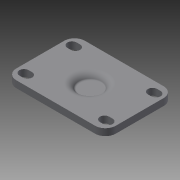
# Autodesk Inventor part: 2SS-TP
Saved by Autodesk Inventor 2014 SP2 (Build 180246200, 246)
## iProperties
Created: 2018-12-09
Part Number: 2SS-TP
Material: Generic
Catalog Web Link: www.cadenas.de
Description: 2 Series Stainless_Steel Top Plate-Capacitiy up to 325 lbs Each
Vendor: COLSONGROUP
Document SubType Name: Modeling
Designer: psadmin
Manufacturer: COLSONGROUP
Mass: 34.703 g
Surface Area: 138.104 cm^2
Volume: 34.703 cm^3
Density: 1 g/cm^3
Appearance: PSOLRGB-175-175-175
Category: PARTsolutions
Company: COLSONGROUP
Title: 2SS-TP
Author: Cadenas PARTsolutions
Comments: Capacitiy up to 325 lbs Each
PSOL_IDENT_0: {$CADENAS_DATA\23d-libs\colsongroup\colson\casters\2_series_stainless_steel\2_series_stainless_steel
PSOL_IDENT_1: _top_plate.prj},180 {VTYP=3D},{NB=2SS-TP},{LINA=2SS-TP},{NN=2 Series Stainless_Steel Top Plate},{DAT
PSOL_IDENT_2: E=13.07.2017 07:15:59},{GEOMDATE=03.02.2017 08:04:00},{VERSION=},{LINEID=40},{WBVAR=},{WBNUMERIC=}
PSOL_IDENT_3: {NB=2SS-TP},{LINA=2SS-TP},{KT=DUMMY},{PN=2SS-TP},{MO=TPS},{HEIGHT=2.50000000},{WIDTH=3.62500000},{HD
PSOL_IDENT_4: Y1=2.81250000},{HDY2=3.06250000},{HDX1=1.75000000},{THK=0.250},{HR=0.170}
NN: 2 Series Stainless_Steel Top Plate
NT: Capacitiy up to 325 lbs Each
NB: 2SS-TP
NBSYN: $PN.
LINA: 2SS-TP
PN: 2SS-TP
MO: TPS
HEIGHT: 2.5
WIDTH: 3.625
HDY1: 2.8125
HDY2: 3.0625
HDX1: 1.75
THK: 0.25
HR: 0.17
SUPPLIER: COLSONGROUP
ARTICLENO: 2SS-TP
BOMINFO: 2SS-TP
CREATOR: CADENAS GmbH
Autodesk Inventor part; units mm, degrees
sketch "Sketch_1" plane through (0, 0, 0) normal (0, 0, 1) x (1, 0, 0)
  line L0 (0, -10.8204) -> (0, -4.4704)
  line L1 (0, -4.4704) -> (9.2111, -4.4704)
  arc A0 (9.2111, -4.4704) -> (10.6049, -3.6564) centre (9.2111, -2.8702) ccw
  arc A1 (16.8656, 0) -> (10.6049, -3.6564) centre (16.8656, -7.1882) ccw
  line L2 (16.8656, 0) -> (25.4, 0)
  line L3 (25.4, 0) -> (25.4, -6.35)
  line L4 (25.4, -6.35) -> (17.3228, -6.35)
  arc A2 (17.3228, -6.35) -> (13.056, -8.1128) centre (17.3228, -12.3952) ccw
  line L5 (13.056, -8.1128) -> (10.8068, -10.3538)
  arc A3 (9.6774, -10.8204) -> (10.8068, -10.3538) centre (9.6774, -9.2202) ccw
  line L6 (9.6774, -10.8204) -> (0, -10.8204)
  line L7 (0, -10.8204) -> (0, -4.4704)
  constraints: 16 end point, 8 point on circle, 4 centre point
revolve "Revolution1" add sketch "Sketch_1" angle 360 about axis through (0, -10.8204, 0) along (0, -1, 0)
sketch "Sketch_2" plane through (0, 0, 0) normal (0, 1, 0) x (-1, 0, 0)
  line L0 (46.0375, 0) -> (25.4, 0)
  arc A0 (-25.4, 0) -> (25.4, 0) centre (0, 0) ccw
  line L1 (-25.4, 0) -> (-46.0375, 0)
  line L2 (-46.0375, 0) -> (-46.0375, -22.225)
  arc A1 (-46.0375, -22.225) -> (-36.5125, -31.75) centre (-36.5125, -22.225) ccw
  line L3 (-36.5125, -31.75) -> (36.5125, -31.75)
  arc A2 (36.5125, -31.75) -> (46.0375, -22.225) centre (36.5125, -22.225) ccw
  line L4 (46.0375, -22.225) -> (46.0375, 0)
  arc A3 (-35.7188, -26.543) -> (-35.7188, -17.907) centre (-35.7187, -22.225) ccw
  line L5 (-35.7188, -17.907) -> (-38.8937, -17.907)
  arc A4 (-38.8937, -17.907) -> (-38.8937, -26.543) centre (-38.8938, -22.225) ccw
  line L6 (-38.8937, -26.543) -> (-35.7188, -26.543)
  arc A5 (38.8937, -26.543) -> (38.8937, -17.907) centre (38.8938, -22.225) ccw
  line L7 (38.8937, -17.907) -> (35.7188, -17.907)
  arc A6 (35.7188, -17.907) -> (35.7188, -26.543) centre (35.7187, -22.225) ccw
  line L8 (35.7188, -26.543) -> (38.8937, -26.543)
  constraints: 18 end point, 14 point on circle, 7 centre point
extrude "Extrusion1" add sketch "Sketch_2" against normal blind 6.35
sketch "Sketch_3" plane through (0, 0, 0) normal (0, 1, 0) x (-1, 0, 0)
  line L0 (46.0375, 0) -> (46.0375, 22.225)
  arc A0 (46.0375, 22.225) -> (36.5125, 31.75) centre (36.5125, 22.225) ccw
  line L1 (36.5125, 31.75) -> (-36.5125, 31.75)
  arc A1 (-36.5125, 31.75) -> (-46.0375, 22.225) centre (-36.5125, 22.225) ccw
  line L2 (-46.0375, 22.225) -> (-46.0375, 0)
  line L3 (-46.0375, 0) -> (-25.4, 0)
  arc A2 (25.4, 0) -> (-25.4, 0) centre (0, 0) ccw
  line L4 (25.4, 0) -> (46.0375, 0)
  arc A3 (-35.7188, 17.907) -> (-35.7188, 26.543) centre (-35.7187, 22.225) ccw
  line L5 (-35.7188, 26.543) -> (-38.8937, 26.543)
  arc A4 (-38.8937, 26.543) -> (-38.8937, 17.907) centre (-38.8938, 22.225) ccw
  line L6 (-38.8937, 17.907) -> (-35.7188, 17.907)
  arc A5 (38.8937, 17.907) -> (38.8937, 26.543) centre (38.8938, 22.225) ccw
  line L7 (38.8937, 26.543) -> (35.7188, 26.543)
  arc A6 (35.7188, 26.543) -> (35.7188, 17.907) centre (35.7187, 22.225) ccw
  line L8 (35.7188, 17.907) -> (38.8937, 17.907)
  constraints: 18 end point, 14 point on circle, 7 centre point
extrude "Extrusion2" add sketch "Sketch_3" against normal blind 6.35
ref_plane "to_rivet_XY" through (0, -4.4704, 0) normal (0, 1, 0) x (1, 0, 0)
ref_plane "to_rivet_YZ" through (0, -4.4704, 0) normal (1, 0, 0) x (0, 0, -1)
ref_plane "to_rivet_ZX" through (0, -4.4704, 0) normal (0, 0, -1) x (0, 1, 0)
ref_plane "to_upper_race_XY" through (0, -6.35, 0) normal (0, 1, 0) x (1, 0, 0)
ref_plane "to_upper_race_YZ" through (0, -6.35, 0) normal (1, 0, 0) x (0, 0, -1)
ref_plane "to_upper_race_ZX" through (0, -6.35, 0) normal (0, 0, -1) x (0, 1, 0)
ref_plane "top_plate_XY" through (0, 0, 0) normal (0, -1, 0) x (1, 0, 0)
ref_plane "top_plate_YZ" through (0, 0, 0) normal (1, 0, 0) x (0, 0, 1)
ref_plane "top_plate_ZX" through (0, 0, 0) normal (0, 0, 1) x (0, -1, 0)
body "Solid1"
